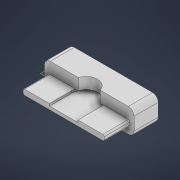
# Autodesk Inventor part: syringe_sledge_fitter
Saved by Autodesk Inventor 2022 (Build 260153000, 153)
## iProperties
Created: 2023-04-24
Part Number: syringe_sledge_fitter
Material: Generic
Document SubType Name: Modeling
Designer: Jakob Saugbjerg
Density: 1 g/cm^3
Appearance: Default
Author: Jakob Saugbjerg
Autodesk Inventor part; units mm, degrees
ref_plane "YZ Plane" through (0, 0, 0) normal (1, 0, 0) x (0, 1, 0)
ref_plane "XZ Plane" through (0, 0, 0) normal (0, 1, 0) x (-1, 0, 0)
ref_plane "XY Plane" through (0, 0, 0) normal (0, 0, 1) x (1, 0, 0)
sketch "Sketch1" plane through (0, 0, 0) normal (0, 0, 1) x (1, 0, 0)
  line L0 (0, 0) -> (63, 0)
  line L1 (63, 0) -> (63, 17)
  line L2 (63, 17) -> (0, 17)
  line L3 (0, 17) -> (0, 0)
  dimension "d0" = 63
  dimension "d1" = 17
  constraints: 8 end point, 2 parallel, 1 horizontal, 1 perpendicular
  measures "d0" distance of L2.end L1.end
  measures "d1" distance of L1.end L0.end
extrude "Extrusion1" add sketch "Sketch1" along normal blind 35
sketch "Sketch2" plane through (0, 17, 0) normal (0, 1, 0) x (1, 0, 0)
  line L0 (63, -35) -> (0, -35) projected
  line L1 (31.5, -35) -> (31.5, -19.25)
  circle A0 centre (31.5, -19.25) radius 8
  line L2 (23.5, -19.25) -> (39.5, -19.25)
  line L3 (39.5, -19.25) -> (39.5, -37.25)
  line L4 (39.5, -37.25) -> (23.5, -37.25)
  line L5 (23.5, -37.25) -> (23.5, -19.25)
  point P0 (0, 0)
  point P1 (23.5, -35)
  point P2 (39.5, -35)
  dimension "d66" = 15.75
  dimension "d67" = 16
  constraints: 10 end point, 2 parallel, 2 point on circle, 1 centre point, 1 coincident, 1 horizontal, 1 midpoint, 1 perpendicular, 1 vertical
  measures "d66" distance of L1.start L1.end
  measures "d67" diameter of A0
extrude "10 mL cross" cut sketch "Sketch2" against normal blind 8 contours L0 L1 A0 L3 | L0 L5 A0 L1 | L2 A0 | A0 L1 L2 | A0 L2 L1
sketch "Sketch3" plane through (0, 9, 0) normal (0, 1, 0) x (1, 0, 0)
  arc A0 (39.5, -19.25) -> (23.5, -19.25) centre (31.5, -19.25) ccw projected
  circle A1 centre (31.5, -19.25) radius 10
  line L0 (21.5, -19.25) -> (41.5, -19.25)
  line L1 (41.5, -19.25) -> (41.5, -35)
  line L2 (41.5, -35) -> (21.5, -35)
  line L3 (21.5, -35) -> (21.5, -19.25)
  point P0 (31.5, -17)
  dimension "d68" = 20
  dimension "d69" = 15.75
  constraints: 8 end point, 2 parallel, 2 point on circle, 1 centre point, 1 coincident, 1 horizontal, 1 perpendicular
  measures "d68" diameter of A1
  measures "d69" distance of L0.end L1.end
extrude "10 mL top" cut sketch "Sketch3" against normal blind 1.5
sketch "Sketch4" plane through (0, 17, 0) normal (0, 1, 0) x (1, 0, 0)
  line L0 (63, -35) -> (0, -35)
  line L1 (0, -35) -> (0, -17)
  line L2 (0, -17) -> (63, -17)
  line L3 (63, -17) -> (63, -35)
  point P0 (0, 0)
  dimension "d19" = 63
  dimension "d20" = 18
  constraints: 8 end point, 2 parallel, 1 horizontal, 1 perpendicular
  measures "d19" distance of L1.end L2.end
  measures "d20" distance of L0.end L1.end
extrude "Extrusion4" cut sketch "Sketch4" against normal blind 8
sketch "Sketch10" plane through (0, 0, 0) normal (0, 0, -1) x (-1, 0, 0)
  line L0 (-19.7584, 8.8263) -> (-18.2714, 8.8263)
  line L1 (-18.2714, 8.8263) -> (-18.2714, 8.515)
  line L2 (-18.2714, 8.515) -> (-18.8247, 8.515)
  line L3 (-18.8247, 8.515) -> (-18.8247, 6.4723)
  line L4 (-18.8247, 6.4723) -> (-18.2714, 6.4723)
  line L5 (-18.2714, 6.4723) -> (-18.2714, 6.1932)
  spline S0 degree 2 poles (-18.2714, 6.1932) (-18.5851, 6.1932) (-18.8815, 6.0154) (-18.9013, 5.7684) knots 0 0 0 1 2 2 2
  line L6 (-18.9013, 5.7684) -> (-19.2174, 5.7684)
  line L7 (-19.2174, 5.7684) -> (-19.2174, 8.515)
  line L8 (-19.2174, 8.515) -> (-19.7584, 8.515)
  line L9 (-19.7584, 8.515) -> (-19.7584, 8.8263)
  spline S1 degree 2 poles (-22.216, 7.3023) (-22.216, 8.1223) (-21.7393, 8.8905) (-21.2428, 8.8905) knots 0 0 0 1 2 2 2
  spline S2 degree 2 poles (-21.2428, 8.8905) (-20.739, 8.8905) (-20.2672, 8.1075) (-20.2672, 7.3047) knots 0 0 0 1 2 2 2
  spline S3 degree 2 poles (-20.2672, 7.3047) (-20.2672, 6.4798) (-20.7439, 5.7165) (-21.2428, 5.7165) knots 0 0 0 1 2 2 2
  spline S4 degree 2 poles (-21.2428, 5.7165) (-21.7443, 5.7165) (-22.216, 6.5069) (-22.216, 7.3023) knots 0 0 0 1 2 2 2
  spline S5 degree 2 poles (-21.6924, 8.231) (-21.7517, 8.0803) (-21.8011, 7.616) (-21.8011, 7.3023) knots 0 0 0 1 2 2 2
  spline S6 degree 2 poles (-21.8011, 7.3023) (-21.8011, 6.9886) (-21.7517, 6.5267) (-21.6899, 6.3711) knots 0 0 0 1 2 2 2
  spline S7 degree 2 poles (-21.6899, 6.3711) (-21.6282, 6.2155) (-21.4133, 6.0549) (-21.2428, 6.0549) knots 0 0 0 1 2 2 2
  spline S8 degree 2 poles (-21.2428, 6.0549) (-21.0724, 6.0549) (-20.8526, 6.2155) (-20.7884, 6.376) knots 0 0 0 1 2 2 2
  spline S9 degree 2 poles (-20.7884, 6.376) (-20.7266, 6.5316) (-20.6822, 7.0059) (-20.6822, 7.3047) knots 0 0 0 1 2 2 2
  spline S10 degree 2 poles (-20.6822, 7.3047) (-20.6822, 7.6258) (-20.7217, 8.0556) (-20.7859, 8.2236) knots 0 0 0 1 2 2 2
  spline S11 degree 2 poles (-20.7859, 8.2236) (-20.8452, 8.3817) (-21.065, 8.5521) (-21.2428, 8.5521) knots 0 0 0 1 2 2 2
  spline S12 degree 2 poles (-21.2428, 8.5521) (-21.4108, 8.5521) (-21.6306, 8.3915) (-21.6924, 8.231) knots 0 0 0 1 2 2 2
  line L10 (-26.5657, 8.8263) -> (-26.5657, 7.5023)
  spline S13 degree 2 poles (-26.5657, 7.5023) (-26.5657, 7.3443) (-26.541, 7.075) (-26.5015, 7.0009) knots 0 0 0 1 2 2 2
  spline S14 degree 2 poles (-26.5015, 7.0009) (-26.462, 6.9194) (-26.3113, 6.8404) (-26.1804, 6.8404) knots 0 0 0 1 2 2 2
  spline S15 degree 2 poles (-26.1804, 6.8404) (-26.0618, 6.8404) (-25.7901, 6.9861) (-25.6469, 7.1244) knots 0 0 0 1 2 2 2
  spline S16 degree 2 poles (-25.6469, 7.1244) (-25.6494, 7.159) (-25.6543, 7.2553) (-25.6543, 7.3196) knots 0 0 0 1 2 2 2
  line L11 (-25.6543, 7.3196) -> (-25.6543, 8.8263)
  line L12 (-25.6543, 8.8263) -> (-25.269, 8.8263)
  line L13 (-25.269, 8.8263) -> (-25.269, 7.5023)
  spline S17 degree 2 poles (-25.269, 7.5023) (-25.269, 7.3443) (-25.2443, 7.075) (-25.2048, 7.0009) knots 0 0 0 1 2 2 2
  spline S18 degree 2 poles (-25.2048, 7.0009) (-25.1652, 6.9194) (-25.0146, 6.8404) (-24.8837, 6.8404) knots 0 0 0 1 2 2 2
  spline S19 degree 2 poles (-24.8837, 6.8404) (-24.7601, 6.8404) (-24.486, 6.996) (-24.3575, 7.117) knots 0 0 0 1 2 2 2
  line L14 (-24.3575, 7.117) -> (-24.3575, 8.8263)
  line L15 (-24.3575, 8.8263) -> (-23.9722, 8.8263)
  line L16 (-23.9722, 8.8263) -> (-23.9722, 6.539)
  line L17 (-23.9722, 6.539) -> (-24.3575, 6.539)
  line L18 (-24.3575, 6.539) -> (-24.3575, 6.791)
  spline S20 degree 2 poles (-24.3575, 6.791) (-24.5082, 6.6403) (-24.8046, 6.4748) (-24.9825, 6.4748) knots 0 0 0 1 2 2 2
  spline S21 degree 2 poles (-24.9825, 6.4748) (-25.185, 6.4748) (-25.4987, 6.6601) (-25.5802, 6.87) knots 0 0 0 1 2 2 2
  spline S22 degree 2 poles (-25.5802, 6.87) (-25.7556, 6.6749) (-26.0865, 6.4748) (-26.2792, 6.4748) knots 0 0 0 1 2 2 2
  spline S23 degree 2 poles (-26.2792, 6.4748) (-26.4274, 6.4748) (-26.6695, 6.5662) (-26.7584, 6.6699) knots 0 0 0 1 2 2 2
  spline S24 degree 2 poles (-26.7584, 6.6699) (-26.8498, 6.7737) (-26.9511, 7.0849) (-26.9511, 7.3196) knots 0 0 0 1 2 2 2
  line L19 (-26.9511, 7.3196) -> (-26.9511, 8.8263)
  line L20 (-26.9511, 8.8263) -> (-26.5657, 8.8263)
  line L21 (-29.2877, 8.8263) -> (-27.5216, 8.8263)
  line L22 (-27.5216, 8.8263) -> (-27.5216, 5.7783)
  line L23 (-27.5216, 5.7783) -> (-27.9267, 5.7783)
  line L24 (-27.9267, 5.7783) -> (-27.9267, 8.4656)
  line L25 (-27.9267, 8.4656) -> (-29.2877, 8.4656)
  line L26 (-29.2877, 8.4656) -> (-29.2877, 8.8263)
  spline S25 degree 2 poles (-31.5033, 8.8806) (-31.2736, 8.8806) (-30.8759, 8.7571) (-30.745, 8.6879) knots 0 0 0 1 2 2 2
  line L27 (-30.745, 8.6879) -> (-30.745, 8.2557)
  line L28 (-30.745, 8.2557) -> (-30.7648, 8.2557)
  spline S26 degree 2 poles (-30.7648, 8.2557) (-30.8142, 8.2952) (-30.9475, 8.3891) (-31.0587, 8.4409) knots 0 0 0 1 2 2 2
  spline S27 degree 2 poles (-31.0587, 8.4409) (-31.155, 8.4879) (-31.3921, 8.557) (-31.5181, 8.557) knots 0 0 0 1 2 2 2
  spline S28 degree 2 poles (-31.5181, 8.557) (-31.6095, 8.557) (-31.8195, 8.515) (-31.8689, 8.4805) knots 0 0 0 1 2 2 2
  spline S29 degree 2 poles (-31.8689, 8.4805) (-31.9405, 8.4335) (-32.0047, 8.3273) (-32.0047, 8.2186) knots 0 0 0 1 2 2 2
  spline S30 degree 2 poles (-32.0047, 8.2186) (-32.0047, 8.0828) (-31.8565, 7.942) (-31.6663, 7.8951) knots 0 0 0 1 2 2 2
  spline S31 degree 2 poles (-31.6663, 7.8951) (-31.5922, 7.8778) (-31.3551, 7.8284) (-31.2538, 7.8012) knots 0 0 0 1 2 2 2
  spline S32 degree 2 poles (-31.2538, 7.8012) (-30.992, 7.7246) (-30.7549, 7.4085) (-30.7549, 7.1837) knots 0 0 0 1 2 2 2
  spline S33 degree 2 poles (-30.7549, 7.1837) (-30.7549, 6.8725) (-31.2217, 6.4847) (-31.607, 6.4847) knots 0 0 0 1 2 2 2
  spline S34 degree 2 poles (-31.607, 6.4847) (-31.7972, 6.4847) (-32.1825, 6.5786) (-32.3135, 6.6502) knots 0 0 0 1 2 2 2
  line L29 (-32.3135, 6.6502) -> (-32.3135, 7.0627)
  line L30 (-32.3135, 7.0627) -> (-32.2937, 7.0627)
  spline S35 degree 2 poles (-32.2937, 7.0627) (-32.1455, 6.9441) (-31.7849, 6.8083) (-31.5996, 6.8083) knots 0 0 0 1 2 2 2
  spline S36 degree 2 poles (-31.5996, 6.8083) (-31.4094, 6.8083) (-31.1476, 6.9688) (-31.1476, 7.1294) knots 0 0 0 1 2 2 2
  spline S37 degree 2 poles (-31.1476, 7.1294) (-31.1476, 7.2751) (-31.3032, 7.4159) (-31.4761, 7.4603) knots 0 0 0 1 2 2 2
  spline S38 degree 2 poles (-31.4761, 7.4603) (-31.5601, 7.4826) (-31.7725, 7.527) (-31.8886, 7.5542) knots 0 0 0 1 2 2 2
  spline S39 degree 2 poles (-31.8886, 7.5542) (-32.1406, 7.6184) (-32.3974, 7.9124) (-32.3974, 8.1668) knots 0 0 0 1 2 2 2
  spline S40 degree 2 poles (-32.3974, 8.1668) (-32.3974, 8.315) (-32.2813, 8.5768) (-32.1677, 8.6731) knots 0 0 0 1 2 2 2
  spline S41 degree 2 poles (-32.1677, 8.6731) (-32.0467, 8.7744) (-31.7379, 8.8806) (-31.5033, 8.8806) knots 0 0 0 1 2 2 2
  line L31 (-34.5513, 6.539) -> (-33.3212, 9.6685)
  line L32 (-33.3212, 9.6685) -> (-32.9087, 9.6685)
  line L33 (-32.9087, 9.6685) -> (-33.3188, 8.7151)
  line L34 (-33.3188, 8.7151) -> (-32.4888, 6.539)
  line L35 (-32.4888, 6.539) -> (-32.9038, 6.539)
  line L36 (-32.9038, 6.539) -> (-33.5287, 8.2335)
  line L37 (-33.5287, 8.2335) -> (-34.1512, 6.539)
  line L38 (-34.1512, 6.539) -> (-34.5513, 6.539)
  line L39 (-36.0555, 6.9515) -> (-36.0358, 6.9515)
  spline S42 degree 2 poles (-36.0358, 6.9515) (-35.9913, 6.9392) (-35.895, 6.9342) (-35.8283, 6.9342) knots 0 0 0 1 2 2 2
  spline S43 degree 2 poles (-35.8283, 6.9342) (-35.6727, 6.9342) (-35.3664, 7.0701) (-35.2281, 7.2035) knots 0 0 0 1 2 2 2
  line L40 (-35.2281, 7.2035) -> (-35.2281, 8.8263)
  line L41 (-35.2281, 8.8263) -> (-34.8428, 8.8263)
  line L42 (-34.8428, 8.8263) -> (-34.8428, 6.539)
  line L43 (-34.8428, 6.539) -> (-35.2281, 6.539)
  line L44 (-35.2281, 6.539) -> (-35.2281, 6.8799)
  spline S44 degree 2 poles (-35.2281, 6.8799) (-35.438, 6.6922) (-35.7517, 6.539) (-35.8999, 6.539) knots 0 0 0 1 2 2 2
  spline S45 degree 2 poles (-35.8999, 6.539) (-35.9592, 6.539) (-36.0185, 6.544) (-36.0555, 6.5514) knots 0 0 0 1 2 2 2
  line L45 (-36.0555, 6.5514) -> (-36.0555, 6.9515)
  line L46 (-36.7471, 8.8263) -> (-36.3618, 8.8263)
  line L47 (-36.3618, 8.8263) -> (-36.3618, 6.539)
  line L48 (-36.3618, 6.539) -> (-36.7471, 6.539)
  line L49 (-36.7471, 6.539) -> (-36.7471, 8.8263)
  line L50 (-36.7743, 6.1586) -> (-36.3371, 6.1586)
  line L51 (-36.3371, 6.1586) -> (-36.3371, 5.7585)
  line L52 (-36.3371, 5.7585) -> (-36.7743, 5.7585)
  line L53 (-36.7743, 5.7585) -> (-36.7743, 6.1586)
  line L54 (-39.1085, 8.8263) -> (-38.7232, 8.8263)
  line L55 (-38.7232, 8.8263) -> (-38.7232, 7.5221)
  spline S46 degree 2 poles (-38.7232, 7.5221) (-38.7232, 7.364) (-38.6935, 7.0923) (-38.6491, 7.0108) knots 0 0 0 1 2 2 2
  spline S47 degree 2 poles (-38.6491, 7.0108) (-38.6021, 6.9244) (-38.4342, 6.8404) (-38.2909, 6.8404) knots 0 0 0 1 2 2 2
  spline S48 degree 2 poles (-38.2909, 6.8404) (-38.1476, 6.8404) (-37.8438, 6.9935) (-37.6981, 7.117) knots 0 0 0 1 2 2 2
  line L56 (-37.6981, 7.117) -> (-37.6981, 8.8263)
  line L57 (-37.6981, 8.8263) -> (-37.3128, 8.8263)
  line L58 (-37.3128, 8.8263) -> (-37.3128, 6.539)
  line L59 (-37.3128, 6.539) -> (-37.6981, 6.539)
  line L60 (-37.6981, 6.539) -> (-37.6981, 6.7934)
  spline S49 degree 2 poles (-37.6981, 6.7934) (-37.871, 6.6378) (-38.2044, 6.4748) (-38.3922, 6.4748) knots 0 0 0 1 2 2 2
  spline S50 degree 2 poles (-38.3922, 6.4748) (-38.7281, 6.4748) (-39.1085, 6.9194) (-39.1085, 7.3418) knots 0 0 0 1 2 2 2
  line L61 (-39.1085, 7.3418) -> (-39.1085, 8.8263)
  spline S51 degree 2 poles (-39.7309, 9.1918) (-39.7704, 9.2091) (-39.9211, 9.2635) (-40.0174, 9.2857) knots 0 0 0 1 2 2 2
  spline S52 degree 2 poles (-40.0174, 9.2857) (-40.1237, 9.3129) (-40.304, 9.345) (-40.4102, 9.345) knots 0 0 0 1 2 2 2
  spline S53 degree 2 poles (-40.4102, 9.345) (-40.588, 9.345) (-40.835, 9.2511) (-40.9042, 9.1671) knots 0 0 0 1 2 2 2
  spline S54 degree 2 poles (-40.9042, 9.1671) (-40.9709, 9.0831) (-41.0227, 8.8633) (-41.0227, 8.7225) knots 0 0 0 1 2 2 2
  line L62 (-41.0227, 8.7225) -> (-41.0227, 8.5225)
  spline S55 degree 2 poles (-41.0227, 8.5225) (-40.8671, 8.6583) (-40.5683, 8.7867) (-40.3435, 8.7867) knots 0 0 0 1 2 2 2
  spline S56 degree 2 poles (-40.3435, 8.7867) (-39.9532, 8.7867) (-39.4913, 8.2063) (-39.4913, 7.6604) knots 0 0 0 1 2 2 2
  spline S57 degree 2 poles (-39.4913, 7.6604) (-39.4913, 7.3764) (-39.6519, 6.9367) (-39.7853, 6.7811) knots 0 0 0 1 2 2 2
  spline S58 degree 2 poles (-39.7853, 6.7811) (-39.9137, 6.6354) (-40.2669, 6.4748) (-40.4546, 6.4748) knots 0 0 0 1 2 2 2
  spline S59 degree 2 poles (-40.4546, 6.4748) (-40.6325, 6.4748) (-40.8918, 6.5588) (-41.0227, 6.6354) knots 0 0 0 1 2 2 2
  line L63 (-41.0227, 6.6354) -> (-41.045, 6.539)
  line L64 (-41.045, 6.539) -> (-41.4081, 6.539)
  line L65 (-41.4081, 6.539) -> (-41.4081, 8.5644)
  spline S60 degree 2 poles (-41.4081, 8.5644) (-41.4081, 9.1474) (-40.9017, 9.6908) (-40.3805, 9.6908) knots 0 0 0 1 2 2 2
  spline S61 degree 2 poles (-40.3805, 9.6908) (-40.2126, 9.6908) (-39.8618, 9.6364) (-39.7112, 9.592) knots 0 0 0 1 2 2 2
  line L66 (-39.7112, 9.592) -> (-39.7112, 9.1918)
  line L67 (-39.7112, 9.1918) -> (-39.7309, 9.1918)
  line L68 (-41.0227, 8.2063) -> (-41.0227, 6.9491)
  spline S62 degree 2 poles (-41.0227, 6.9491) (-40.8795, 6.8799) (-40.6374, 6.8206) (-40.5164, 6.8206) knots 0 0 0 1 2 2 2
  spline S63 degree 2 poles (-40.5164, 6.8206) (-40.2249, 6.8206) (-39.889, 7.2504) (-39.889, 7.653) knots 0 0 0 1 2 2 2
  spline S64 degree 2 poles (-39.889, 7.653) (-39.889, 8.0334) (-40.1434, 8.4311) (-40.4299, 8.4311) knots 0 0 0 1 2 2 2
  spline S65 degree 2 poles (-40.4299, 8.4311) (-40.5806, 8.4311) (-40.8968, 8.3125) (-41.0227, 8.2063) knots 0 0 0 1 2 2 2
  spline S66 degree 2 poles (-42.9592, 8.8781) (-42.4109, 8.8781) (-41.8082, 8.2631) (-41.8082, 7.695) knots 0 0 0 1 2 2 2
  spline S67 degree 2 poles (-41.8082, 7.695) (-41.8082, 7.1368) (-42.3936, 6.4748) (-42.8654, 6.4748) knots 0 0 0 1 2 2 2
  spline S68 degree 2 poles (-42.8654, 6.4748) (-43.0778, 6.4748) (-43.4063, 6.5983) (-43.5273, 6.7292) knots 0 0 0 1 2 2 2
  spline S69 degree 2 poles (-43.5273, 6.7292) (-43.6508, 6.8601) (-43.7817, 7.238) (-43.7817, 7.5122) knots 0 0 0 1 2 2 2
  line L69 (-43.7817, 7.5122) -> (-43.7817, 7.7222)
  line L70 (-43.7817, 7.7222) -> (-42.1985, 7.7222)
  spline S70 degree 2 poles (-42.1985, 7.7222) (-42.1985, 8.1198) (-42.5986, 8.5422) (-42.9543, 8.5422) knots 0 0 0 1 2 2 2
  spline S71 degree 2 poles (-42.9543, 8.5422) (-43.0803, 8.5422) (-43.3248, 8.4854) (-43.4236, 8.4409) knots 0 0 0 1 2 2 2
  spline S72 degree 2 poles (-43.4236, 8.4409) (-43.5273, 8.3915) (-43.6706, 8.3051) (-43.7175, 8.2656) knots 0 0 0 1 2 2 2
  line L71 (-43.7175, 8.2656) -> (-43.7398, 8.2656)
  line L72 (-43.7398, 8.2656) -> (-43.7398, 8.6855)
  spline S73 degree 2 poles (-43.7398, 8.6855) (-43.6731, 8.7126) (-43.4705, 8.7917) (-43.3915, 8.8139) knots 0 0 0 1 2 2 2
  spline S74 degree 2 poles (-43.3915, 8.8139) (-43.2803, 8.846) (-43.0976, 8.8781) (-42.9592, 8.8781) knots 0 0 0 1 2 2 2
  spline S75 degree 2 poles (-43.4063, 7.4282) (-43.4014, 7.2726) (-43.3371, 7.0454) (-43.2754, 6.9688) knots 0 0 0 1 2 2 2
  spline S76 degree 2 poles (-43.2754, 6.9688) (-43.2087, 6.8824) (-42.9987, 6.791) (-42.8431, 6.791) knots 0 0 0 1 2 2 2
  spline S77 degree 2 poles (-42.8431, 6.791) (-42.69, 6.791) (-42.4751, 6.8824) (-42.3862, 6.9713) knots 0 0 0 1 2 2 2
  spline S78 degree 2 poles (-42.3862, 6.9713) (-42.2997, 7.0627) (-42.2108, 7.2825) (-42.1985, 7.4282) knots 0 0 0 1 2 2 2
  line L73 (-42.1985, 7.4282) -> (-43.4063, 7.4282)
  point P0 (0, 0)
  point P1 (-17.8095, 5.7165)
  dimension "d3" = 0
  constraints: 1 other
emboss "Emboss1" sketch "Sketch10" operation cut depth 1 direction (0, 0, 1)
ref_plane "Work Plane1" through (2, 0, 0) normal (0, -1, 0) x (1, 0, 0)
sketch "Sketch11" plane through (2, 0, 0) normal (0, -1, 0) x (1, 0, 0)
  line L0 (-2, 35) -> (-2, 0) projected
  line L1 (61, 17) -> (61, 35) projected
  line L2 (-2, 35) -> (61, 35)
  line L3 (61, 35) -> (61, 17)
  line L4 (61, 17) -> (-2, 17)
  line L5 (-2, 17) -> (-2, 35)
  point P0 (-2, 17)
  dimension "d41" = 18
  constraints: 8 end point, 2 parallel, 1 horizontal, 1 perpendicular
  measures "d41" distance of L2.end L1.start
extrude "Extrusion8" cut sketch "Sketch11" against normal blind 5.2
sketch "Sketch13" plane through (0, 0, 35) normal (0, 0, 1) x (1, 0, 0)
  line L0 (63, 3.2) -> (0, 3.2) projected
  line L1 (0, 9) -> (63, 9) projected
  line L2 (0, 3.2) -> (3, 3.2)
  line L3 (3, 3.2) -> (3, 9)
  line L4 (3, 9) -> (0, 9)
  line L5 (0, 9) -> (0, 3.2)
  line L6 (63, 9) -> (0, 9) projected
  line L7 (63, 9) -> (60, 9)
  line L8 (60, 9) -> (60, 3.2)
  line L9 (60, 3.2) -> (63, 3.2)
  line L10 (63, 3.2) -> (63, 9)
  point P0 (0, 0)
  point P1 (19, 7)
  point P2 (41.1047, 7)
  point P3 (60, 9)
  point P4 (60, 3.2)
  point P5 (0, 9)
  dimension "d52" = 3
  dimension "d53" = 3
  constraints: 16 end point, 4 parallel, 2 horizontal, 2 perpendicular, 1 point on line, 3 other
  measures "d52" distance of L4.end L3.end
  measures "d53" distance of L9.end L8.end
extrude "Extrusion10" cut sketch "Sketch13" against normal blind 18 contours L0 L8 L1 L10 | L0 L5 L1 L3
fillet "Fillet5" radius 1 4 edges at (3, 9, 26) (60, 9, 26) (3, 5.2, 26) (60, 5.2, 26)
fillet "Fillet6" radius 4 4 edges at (63, 17, 8.5) (63, 0, 8.5) (0, 17, 8.5) (0, 0, 8.5)
body "Solid1"
